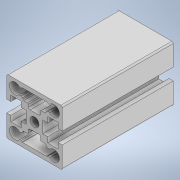
# Autodesk Inventor part: AFSW-2020-4
Saved by Autodesk Inventor 2021 (Build 250183000, 183)
## iProperties
Created: 2021-04-18
Part Number: AFSW-2020-4
Material: 一般
Document SubType Name: Modeling
Designer: gisen
Density: 1 g/cm^3
Appearance: 既定
Sending System: Autodesk Inventor 2014
MC: AMD64
MC_MODEL: Intel64 Family 6 Model 94 Stepping 3, GenuineIntel
OS: Windows_NT
OS_RELEASE: 6.1
FRU: Autodesk
FORMAT: text
GUISE: transmit
KEY: AFSW-2020-4
FILE: C:\Users\AMS43\Documents\Inventor\AMS\Inventorì¬f\parasolidf\AFSW-2020-4.x_t
DATE: Mon, 29 Aug 2016 10:08:56 GMT
Author: gisen
Autodesk Inventor part; units mm, degrees
ref_plane "YZ Plane" through (0, 0, 0) normal (1, 0, 0) x (0, 1, 0)
ref_plane "XZ Plane" through (0, 0, 0) normal (0, 1, 0) x (-1, 0, 0)
ref_plane "作業平面1" through (-9.5, -10, 1000) normal (0, 0, 1) x (1, 0, 0)
sketch "スケッチ1" plane through (-9.5, -10, 1000) normal (0, 0, 1) x (1, 0, 0)
  line L0 (-0.5, 12.15) -> (1, 12.15) projected
  line L1 (1, 12.15) -> (1, 14.15) projected
  line L2 (1, 14.15) -> (4.7, 14.15) projected
  line L3 (4.7, 14.15) -> (4.7, 12.15) projected
  line L4 (4.7, 12.15) -> (6.5, 12.15) projected
  line L5 (6.5, 12.15) -> (6.5, 7.85) projected
  line L6 (6.5, 7.85) -> (4.7, 7.85) projected
  line L7 (4.7, 7.85) -> (4.7, 5.85) projected
  line L8 (4.7, 5.85) -> (1, 5.85) projected
  line L9 (1, 5.85) -> (1, 7.85) projected
  line L10 (1, 7.85) -> (-0.5, 7.85) projected
  line L11 (-0.5, 7.85) -> (-0.5, 0.5) projected
  arc A0 (-0.5, 0.5) -> (0, 0) centre (0, 0.5) ccw projected
  line L12 (0, 0) -> (19, 0) projected
  arc A1 (19, 0) -> (19.5, 0.5) centre (19, 0.5) ccw projected
  line L13 (19.5, 0.5) -> (19.5, 7.85) projected
  line L14 (19.5, 7.85) -> (18, 7.85) projected
  line L15 (18, 7.85) -> (18, 5.85) projected
  line L16 (18, 5.85) -> (14.3, 5.85) projected
  line L17 (14.3, 5.85) -> (14.3, 7.85) projected
  line L18 (14.3, 7.85) -> (12.5, 7.85) projected
  line L19 (12.5, 7.85) -> (12.5, 12.15) projected
  line L20 (12.5, 12.15) -> (14.3, 12.15) projected
  line L21 (14.3, 12.15) -> (14.3, 14.15) projected
  line L22 (14.3, 14.15) -> (18, 14.15) projected
  line L23 (18, 14.15) -> (18, 12.15) projected
  line L24 (18, 12.15) -> (19.5, 12.15) projected
  line L25 (19.5, 12.15) -> (19.5, 19.5) projected
  arc A2 (19.5, 19.5) -> (19, 20) centre (19, 19.5) ccw projected
  line L26 (19, 20) -> (0, 20) projected
  arc A3 (0, 20) -> (-0.5, 19.5) centre (0, 19.5) ccw projected
  line L27 (-0.5, 19.5) -> (-0.5, 12.15) projected
  line L28 (13.65, 15.1813) -> (13.65, 15.1) projected
  arc A4 (13.35, 14.8) -> (13.65, 15.1) centre (13.35, 15.1) ccw projected
  line L29 (13.35, 14.8) -> (11.95, 14.8) projected
  arc A5 (11.95, 14.8) -> (11.65, 14.5) centre (11.95, 14.5) ccw projected
  line L30 (11.65, 14.5) -> (11.65, 13.6) projected
  arc A6 (11.05, 13) -> (11.65, 13.6) centre (11.05, 13.6) ccw projected
  line L31 (11.05, 13) -> (7.9486, 13) projected
  arc A7 (7.3486, 13.5976) -> (7.9486, 13) centre (7.9486, 13.6) ccw projected
  line L32 (7.3486, 13.5976) -> (7.3486, 14.4976) projected
  arc A8 (7.3486, 14.4976) -> (7.0486, 14.7976) centre (7.0486, 14.4976) ccw projected
  line L33 (7.0486, 14.7976) -> (5.6486, 14.7976) projected
  arc A9 (5.3486, 15.0976) -> (5.6486, 14.7976) centre (5.6486, 15.0976) ccw projected
  arc A10 (5.3486, 15.0976) -> (5.2091, 15.4359) centre (5.0591, 15.1761) ccw projected
  line L34 (5.2091, 15.4359) -> (4.6213, 15.7753) projected
  arc A11 (4.6213, 15.7753) -> (3.9971, 15.6738) centre (4.3713, 15.3422) ccw projected
  arc A12 (3.9971, 18.3262) -> (3.9971, 15.6738) centre (2.5, 17) ccw projected
  arc A13 (3.9971, 18.3262) -> (4.6213, 18.2247) centre (4.3713, 18.6578) ccw projected
  line L35 (4.6213, 18.2247) -> (5.0285, 18.4598) projected
  arc A14 (5.1785, 18.5) -> (5.0285, 18.4598) centre (5.1785, 18.2) ccw projected
  line L36 (5.1785, 18.5) -> (13.8215, 18.5) projected
  arc A15 (13.9715, 18.4598) -> (13.8215, 18.5) centre (13.8215, 18.2) ccw projected
  line L37 (13.9715, 18.4598) -> (14.3787, 18.2247) projected
  arc A16 (14.3787, 18.2247) -> (15.0029, 18.3262) centre (14.6287, 18.6578) ccw projected
  arc A17 (15.0029, 15.6738) -> (15.0029, 18.3262) centre (16.5, 17) ccw projected
  arc A18 (15.0029, 15.6738) -> (14.3787, 15.7753) centre (14.6287, 15.3422) ccw projected
  line L38 (14.3787, 15.7753) -> (13.8, 15.4412) projected
  arc A19 (13.8, 15.4412) -> (13.65, 15.1813) centre (13.95, 15.1813) ccw projected
  arc A20 (11.65, 6.4) -> (11.05, 7) centre (11.05, 6.4) ccw projected
  line L39 (11.65, 6.4) -> (11.65, 5.5) projected
  arc A21 (11.65, 5.5) -> (11.95, 5.2) centre (11.95, 5.5) ccw projected
  line L40 (11.95, 5.2) -> (13.35, 5.2) projected
  arc A22 (13.65, 4.9) -> (13.35, 5.2) centre (13.35, 4.9) ccw projected
  arc A23 (13.65, 4.9) -> (13.7909, 4.5641) centre (13.9403, 4.8243) ccw projected
  line L41 (13.7909, 4.5641) -> (14.3787, 4.2247) projected
  arc A24 (14.3787, 4.2247) -> (15.0029, 4.3262) centre (14.6287, 4.6578) ccw projected
  arc A25 (15.0029, 1.6738) -> (15.0029, 4.3262) centre (16.5, 3) ccw projected
  arc A26 (15.0029, 1.6738) -> (14.3787, 1.7753) centre (14.6287, 1.3422) ccw projected
  line L42 (14.3787, 1.7753) -> (13.9715, 1.5402) projected
  arc A27 (13.8215, 1.5) -> (13.9715, 1.5402) centre (13.8215, 1.8) ccw projected
  line L43 (13.8215, 1.5) -> (5.1785, 1.5) projected
  arc A28 (5.0285, 1.5402) -> (5.1785, 1.5) centre (5.1785, 1.8) ccw projected
  line L44 (5.0285, 1.5402) -> (4.6213, 1.7753) projected
  arc A29 (4.6213, 1.7753) -> (3.9971, 1.6738) centre (4.3713, 1.3422) ccw projected
  arc A30 (3.9971, 4.3262) -> (3.9971, 1.6738) centre (2.5, 3) ccw projected
  arc A31 (3.9971, 4.3262) -> (4.6213, 4.2247) centre (4.3713, 4.6578) ccw projected
  line L45 (4.6213, 4.2247) -> (5.2, 4.5588) projected
  arc A32 (5.2, 4.5588) -> (5.35, 4.8187) centre (5.05, 4.8187) ccw projected
  arc A33 (5.6395, 5.1972) -> (5.35, 4.8187) centre (5.6395, 4.8972) ccw projected
  line L46 (5.6395, 5.1972) -> (7.05, 5.1972) projected
  arc A34 (7.05, 5.1972) -> (7.35, 5.4972) centre (7.05, 5.4972) ccw projected
  line L47 (7.35, 5.4972) -> (7.35, 6.4) projected
  arc A35 (7.95, 7) -> (7.35, 6.4) centre (7.95, 6.4) ccw projected
  line L48 (7.95, 7) -> (11.05, 7) projected
  circle A36 centre (9.5, 10) radius 1.65 projected
extrude "押し出し1" add sketch "スケッチ1" along normal blind 40
